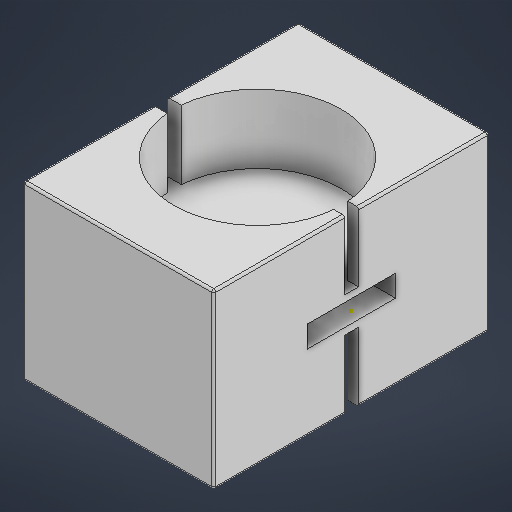
# Autodesk Inventor part: Base_Casing_A0645_v2
Saved by Autodesk Inventor 2026.1 (Build 301233020, 233B)
## iProperties
Created: 2025-09-05
Part Number: Base_Casing_A0645_v2
Material: Generic
Document SubType Name: Modeling
Designer: usman
Density: 1 g/cm^3
Appearance: Default
Author: usman
Autodesk Inventor part; units mm, degrees
ref_plane "YZ Plane" through (0, 0, 0) normal (1, 0, 0) x (0, 1, 0)
ref_plane "XZ Plane" through (0, 0, 0) normal (0, 1, 0) x (-1, 0, 0)
ref_plane "XY Plane" through (0, 0, 0) normal (0, 0, 1) x (1, 0, 0)
sketch "Sketch1" plane through (0, 0, 0) normal (1, 0, 0) x (0, 1, 0)
  line L0 (-39.75, 63.5) -> (39.75, 63.5)
  line L1 (39.75, 63.5) -> (39.75, -63.5)
  line L2 (39.75, -63.5) -> (-39.75, -63.5)
  line L3 (-39.75, -63.5) -> (-39.75, 63.5)
  line L4 (-39.75, 63.5) -> (39.75, -63.5) construction
  line L5 (39.75, 63.5) -> (-39.75, -63.5) construction
  point P0 (0, 0)
  dimension "d0" = 79.5
  constraints: 12 end point, 2 midpoint, 2 parallel, 1 horizontal, 1 perpendicular
  measures "d0" distance of L1.end L2.end
extrude "Extrusion1" add sketch "Sketch1" along normal blind 88
sketch "Sketch2" plane through (88, 0, 0) normal (1, 0, 0) x (0, 0, -1)
  line L0 (-20.32, -5) -> (20.32, -5)
  line L1 (20.32, -5) -> (20.32, 5)
  line L2 (20.32, 5) -> (-20.32, 5)
  line L3 (-20.32, 5) -> (-20.32, -5)
  line L4 (-20.32, -5) -> (20.32, 5) construction
  line L5 (20.32, -5) -> (-20.32, 5) construction
  point P0 (0, 0)
  dimension "d4" = 10
  dimension "d5" = 40.64
  constraints: 12 end point, 2 midpoint, 2 parallel, 1 horizontal, 1 perpendicular
  measures "d4" distance of L0.end L1.end
  measures "d5" distance of L1.end L2.end
extrude "Extrusion2" cut sketch "Sketch2" against normal through all
sketch "Sketch3" plane through (88, 0, 0) normal (1, 0, 0) x (0, 0, -1)
  point P0 (0, 0)
sketch "Sketch4" plane through (0, 39.75, 63.5) normal (0, 1, 0) x (1, 0, 0)
  line L0 (82.3836, 27.6051) -> (7, 99.3949) construction
  line L1 (7, 27.6051) -> (82.3836, 99.3949) construction
  line L2 (0, 127) -> (0, 0) projected
  line L3 (0, 127) -> (88, 127) projected
  circle A0 centre (44.6918, 63.5) radius 38.5
  point P0 (0, 63.5)
  dimension "d23" = 77
  dimension "d24" = 127
  dimension "d25" = 63.5
  constraints: 4 end point, 2 midpoint, 1 centre point, 1 coincident
  measures "d23" diameter of A0
  measures "d24" distance of L2.start L2.end
  measures "d25" vertical distance of point (44.692, 63.5) L2.end
extrude "Extrusion3" cut sketch "Sketch4" against normal blind 31.7
mirror "Mirror1" about plane through (0, 0, 0) normal (0, 1, 0) of "Extrusion3"
sketch "Sketch5" plane through (0, 0, 0) normal (-1, 0, 0) x (0, 0, 1)
  line L0 (-63.5, 39.75) -> (63.5, 39.75) projected
  line L1 (-3.25, 8.05) -> (3.25, 8.05)
  line L2 (3.25, 8.05) -> (3.25, 39.75)
  line L3 (3.25, 39.75) -> (-3.25, 39.75)
  line L4 (-3.25, 39.75) -> (-3.25, 8.05)
  line L5 (-3.25, 8.05) -> (3.25, 39.75) construction
  line L6 (3.25, 8.05) -> (-3.25, 39.75) construction
  point P0 (0, 0)
  point P1 (0, 23.9)
  point P2 (-3.25, 39.75)
  dimension "d12" = 3.25
  dimension "d13" = 31.7
  constraints: 12 end point, 2 midpoint, 2 parallel, 1 horizontal, 1 perpendicular, 1 point on line
  measures "d12" distance from line of point (0, 23.9) L2
  measures "d13" distance of L1.end L2.end
extrude "Extrusion4" cut sketch "Sketch5" against normal through all
mirror "Mirror2" about plane through (0, 0, 0) normal (0, 1, 0) of "Extrusion4"
sketch "Sketch6" plane through (0, 0, 0) normal (-1, 0, 0) x (0, 0, 1)
  line L0 (-53.1221, 38.1768) -> (-13.6279, 38.1768) construction
  line L1 (-13.6279, 38.1768) -> (-13.6279, 7.4202) construction
  line L2 (-13.6279, 7.4202) -> (-53.1221, 7.4202) construction
  line L3 (-53.1221, 7.4202) -> (-53.1221, 38.1768) construction
  line L4 (-63.5, 39.75) -> (-3.25, 39.75) projected
  line L5 (-42.524, 25.8134) -> (-42.524, 31.9094)
  line L6 (-42.524, 31.9094) -> (-41.5692, 31.9094)
  spline S0 degree 2 poles (-41.5692, 31.9094) (-40.7349, 31.9094) (-40.348, 31.8039) knots 0 0 0 1 1 1
  spline S1 degree 2 poles (-40.348, 31.8039) (-39.8052, 31.6581) (-39.1569, 30.8691) (-39.1569, 30.3364) knots 0 0 0 1 2 2 2
  spline S2 degree 2 poles (-39.1569, 30.3364) (-39.1569, 29.9846) (-39.4484, 29.4167) (-39.7801, 29.1705) knots 0 0 0 1 2 2 2
  spline S3 degree 2 poles (-39.7801, 29.1705) (-39.2222, 28.9091) (-38.7096, 28.1252) (-38.7096, 27.5924) knots 0 0 0 1 2 2 2
  spline S4 degree 2 poles (-38.7096, 27.5924) (-38.7096, 27.0748) (-39.2423, 26.2305) (-40.0766, 25.8134) (-40.8153, 25.8134) knots 0 0 0 1 2 3 3 3
  line L7 (-40.8153, 25.8134) -> (-42.524, 25.8134)
  line L8 (-41.3631, 28.482) -> (-41.3631, 26.919)
  line L9 (-41.3631, 26.919) -> (-41.0716, 26.919)
  spline S5 degree 2 poles (-41.0716, 26.919) (-40.353, 26.919) (-39.8504, 27.2859) (-39.8504, 27.6327) knots 0 0 0 1 2 2 2
  spline S6 degree 2 poles (-39.8504, 27.6327) (-39.8504, 28.0246) (-40.4384, 28.482) (-41.1219, 28.482) knots 0 0 0 1 2 2 2
  line L10 (-41.1219, 28.482) -> (-41.3631, 28.482)
  line L11 (-41.3631, 30.8038) -> (-41.3631, 29.5172)
  line L12 (-41.3631, 29.5172) -> (-41.1118, 29.5172)
  spline S7 degree 2 poles (-41.1118, 29.5172) (-40.6897, 29.5172) (-40.2776, 29.8741) (-40.2776, 30.1806) knots 0 0 0 1 2 2 2
  spline S8 degree 2 poles (-40.2776, 30.1806) (-40.2776, 30.4671) (-40.6646, 30.8038) (-41.0666, 30.8038) knots 0 0 0 1 2 2 2
  line L13 (-41.0666, 30.8038) -> (-41.3631, 30.8038)
  line L14 (-34.3977, 30.3213) -> (-33.267, 30.3213)
  line L15 (-33.267, 30.3213) -> (-33.267, 25.8134)
  line L16 (-33.267, 25.8134) -> (-34.3977, 25.8134)
  line L17 (-34.3977, 25.8134) -> (-34.3977, 26.2908)
  spline S9 degree 2 poles (-34.3977, 26.2908) (-34.7294, 25.9742) (-35.3928, 25.6978) (-35.7848, 25.6978) knots 0 0 0 1 2 2 2
  spline S10 degree 2 poles (-35.7848, 25.6978) (-36.6542, 25.6978) (-37.9307, 27.0547) (-37.9307, 28.0598) knots 0 0 0 1 2 2 2
  spline S11 degree 2 poles (-37.9307, 28.0598) (-37.9307, 29.1051) (-36.6994, 30.4369) (-35.8149, 30.4369) knots 0 0 0 1 2 2 2
  spline S12 degree 2 poles (-35.8149, 30.4369) (-35.4129, 30.4369) (-34.6992, 30.1304) (-34.3977, 29.8238) knots 0 0 0 1 2 2 2
  line L18 (-34.3977, 29.8238) -> (-34.3977, 30.3213)
  spline S13 degree 2 poles (-35.5888, 29.3916) (-36.1114, 29.3916) (-36.8049, 28.6528) (-36.8049, 28.0699) knots 0 0 0 1 2 2 2
  spline S14 degree 2 poles (-36.8049, 28.0699) (-36.8049, 27.4869) (-36.0963, 26.7331) (-35.5837, 26.7331) knots 0 0 0 1 2 2 2
  spline S15 degree 2 poles (-35.5837, 26.7331) (-35.051, 26.7331) (-34.3474, 27.4769) (-34.3474, 28.0749) knots 0 0 0 1 2 2 2
  spline S16 degree 2 poles (-34.3474, 28.0749) (-34.3474, 28.6629) (-35.051, 29.3916) (-35.5888, 29.3916) knots 0 0 0 1 2 2 2
  line L19 (-29.3671, 29.6881) -> (-30.0657, 28.9896)
  spline S17 degree 2 poles (-30.0657, 28.9896) (-30.4878, 29.4117) (-30.8346, 29.4117) knots 0 0 0 1 1 1
  spline S18 degree 2 poles (-30.8346, 29.4117) (-31.0256, 29.4117) (-31.2417, 29.2509) (-31.2417, 29.1303) knots 0 0 0 1 2 2 2
  spline S19 degree 2 poles (-31.2417, 29.1303) (-31.2417, 29.0398) (-31.106, 28.884) (-30.8346, 28.7534) knots 0 0 0 1 2 2 2
  line L20 (-30.8346, 28.7534) -> (-30.4225, 28.5473)
  spline S20 degree 2 poles (-30.4225, 28.5473) (-29.7692, 28.2257) (-29.2817, 27.5522) (-29.2817, 27.0999) knots 0 0 0 1 2 2 2
  spline S21 degree 2 poles (-29.2817, 27.0999) (-29.2817, 26.5019) (-30.1612, 25.6978) (-30.9049, 25.6978) knots 0 0 0 1 2 2 2
  spline S22 degree 2 poles (-30.9049, 25.6978) (-31.8899, 25.6978) (-32.4779, 26.4667) knots 0 0 0 1 1 1
  line L21 (-32.4779, 26.4667) -> (-31.7844, 27.2256)
  spline S23 degree 2 poles (-31.7844, 27.2256) (-31.5834, 26.9944) (-31.0507, 26.708) (-30.8446, 26.708) knots 0 0 0 1 2 2 2
  spline S24 degree 2 poles (-30.8446, 26.708) (-30.6185, 26.708) (-30.3471, 26.924) (-30.3471, 27.0648) knots 0 0 0 1 2 2 2
  spline S25 degree 2 poles (-30.3471, 27.0648) (-30.3471, 27.3261) (-30.8396, 27.5723) knots 0 0 0 1 1 1
  line L22 (-30.8396, 27.5723) -> (-31.2215, 27.7633)
  spline S26 degree 2 poles (-31.2215, 27.7633) (-32.3121, 28.3161) (-32.3121, 29.1453) knots 0 0 0 1 1 1
  spline S27 degree 2 poles (-32.3121, 29.1453) (-32.3121, 29.6781) (-31.4879, 30.4369) (-30.8497, 30.4369) knots 0 0 0 1 2 2 2
  spline S28 degree 2 poles (-30.8497, 30.4369) (-30.4074, 30.4369) (-29.6335, 30.0499) (-29.3671, 29.6881) knots 0 0 0 1 2 2 2
  line L23 (-23.8742, 27.7432) -> (-27.5026, 27.7432)
  spline S29 degree 2 poles (-27.5026, 27.7432) (-27.4222, 27.2608) (-26.7388, 26.6929) (-26.2111, 26.6929) knots 0 0 0 1 2 2 2
  spline S30 degree 2 poles (-26.2111, 26.6929) (-25.5778, 26.6929) (-25.1205, 27.1351) knots 0 0 0 1 1 1
  line L24 (-25.1205, 27.1351) -> (-24.1707, 26.6878)
  spline S31 degree 2 poles (-24.1707, 26.6878) (-24.5275, 26.1853) (-25.5226, 25.6978) (-26.206, 25.6978) knots 0 0 0 1 2 2 2
  spline S32 degree 2 poles (-26.206, 25.6978) (-27.2664, 25.6978) (-28.5982, 27.0346) (-28.5982, 28.0447) knots 0 0 0 1 2 2 2
  spline S33 degree 2 poles (-28.5982, 28.0447) (-28.5982, 29.075) (-27.2664, 30.4369) (-26.2664, 30.4369) knots 0 0 0 1 2 2 2
  spline S34 degree 2 poles (-26.2664, 30.4369) (-25.2009, 30.4369) (-23.8692, 29.075) (-23.8692, 27.9593) knots 0 0 0 1 2 2 2
  line L25 (-23.8692, 27.9593) -> (-23.8742, 27.7432)
  spline S35 degree 2 poles (-25.0049, 28.6327) (-25.1155, 29.0097) (-25.7738, 29.477) (-26.2111, 29.477) knots 0 0 0 1 2 2 2
  spline S36 degree 2 poles (-26.2111, 29.477) (-26.6835, 29.477) (-27.0403, 29.2157) knots 0 0 0 1 1 1
  spline S37 degree 2 poles (-27.0403, 29.2157) (-27.2614, 29.0499) (-27.4524, 28.6327) knots 0 0 0 1 1 1
  line L26 (-27.4524, 28.6327) -> (-25.0049, 28.6327)
  line L27 (-48.0471, 21.5476) -> (-46.9214, 21.5476)
  line L28 (-46.9214, 21.5476) -> (-45.5042, 17.296)
  line L29 (-45.5042, 17.296) -> (-44.0769, 21.5476)
  line L30 (-44.0769, 21.5476) -> (-42.9512, 21.5476)
  line L31 (-42.9512, 21.5476) -> (-41.931, 15.4516)
  line L32 (-41.931, 15.4516) -> (-43.0517, 15.4516)
  line L33 (-43.0517, 15.4516) -> (-43.7, 19.3012)
  line L34 (-43.7, 19.3012) -> (-44.9966, 15.4516)
  line L35 (-44.9966, 15.4516) -> (-46.0218, 15.4516)
  line L36 (-46.0218, 15.4516) -> (-47.3033, 19.3012)
  line L37 (-47.3033, 19.3012) -> (-47.9717, 15.4516)
  line L38 (-47.9717, 15.4516) -> (-49.1025, 15.4516)
  line L39 (-49.1025, 15.4516) -> (-48.0471, 21.5476)
  line L40 (-37.795, 19.9595) -> (-36.6642, 19.9595)
  line L41 (-36.6642, 19.9595) -> (-36.6642, 15.4516)
  line L42 (-36.6642, 15.4516) -> (-37.795, 15.4516)
  line L43 (-37.795, 15.4516) -> (-37.795, 15.929)
  spline S38 degree 2 poles (-37.795, 15.929) (-38.1267, 15.6124) (-38.79, 15.336) (-39.182, 15.336) knots 0 0 0 1 2 2 2
  spline S39 degree 2 poles (-39.182, 15.336) (-40.0515, 15.336) (-41.3279, 16.6929) (-41.3279, 17.698) knots 0 0 0 1 2 2 2
  spline S40 degree 2 poles (-41.3279, 17.698) (-41.3279, 18.7433) (-40.0967, 20.0751) (-39.2122, 20.0751) knots 0 0 0 1 2 2 2
  spline S41 degree 2 poles (-39.2122, 20.0751) (-38.8101, 20.0751) (-38.0965, 19.7685) (-37.795, 19.462) knots 0 0 0 1 2 2 2
  line L44 (-37.795, 19.462) -> (-37.795, 19.9595)
  spline S42 degree 2 poles (-38.986, 19.0298) (-39.5087, 19.0298) (-40.2022, 18.291) (-40.2022, 17.7081) knots 0 0 0 1 2 2 2
  spline S43 degree 2 poles (-40.2022, 17.7081) (-40.2022, 17.1251) (-39.4936, 16.3713) (-38.981, 16.3713) knots 0 0 0 1 2 2 2
  spline S44 degree 2 poles (-38.981, 16.3713) (-38.4483, 16.3713) (-37.7447, 17.115) (-37.7447, 17.7131) knots 0 0 0 1 2 2 2
  spline S45 degree 2 poles (-37.7447, 17.7131) (-37.7447, 18.3011) (-38.4483, 19.0298) (-38.986, 19.0298) knots 0 0 0 1 2 2 2
  line L45 (-32.1915, 19.9595) -> (-31.0607, 19.9595)
  line L46 (-31.0607, 19.9595) -> (-31.0607, 16.0999)
  spline S46 degree 2 poles (-31.0607, 16.0999) (-31.0607, 14.9541) (-31.5231, 14.4163) knots 0 0 0 1 1 1
  spline S47 degree 2 poles (-31.5231, 14.4163) (-32.1362, 13.6876) (-33.3825, 13.6876) knots 0 0 0 1 1 1
  spline S48 degree 2 poles (-33.3825, 13.6876) (-34.0459, 13.6876) (-34.9455, 14.0193) (-35.5687, 14.6626) (-35.7194, 15.1199) knots 0 0 0 1 2 3 3 3
  line L47 (-35.7194, 15.1199) -> (-34.4731, 15.1199)
  spline S49 degree 2 poles (-34.4731, 15.1199) (-34.3072, 14.9289) (-33.7846, 14.738) (-33.4278, 14.738) knots 0 0 0 1 2 2 2
  spline S50 degree 2 poles (-33.4278, 14.738) (-32.9755, 14.738) (-32.4176, 15.0194) (-32.1915, 15.4667) (-32.1915, 16.0145) knots 0 0 0 1 2 3 3 3
  spline S51 degree 2 poles (-32.1915, 16.0145) (-32.488, 15.7129) (-33.1413, 15.4516) (-33.5584, 15.4516) knots 0 0 0 1 2 2 2
  spline S52 degree 2 poles (-33.5584, 15.4516) (-34.463, 15.4516) (-35.7144, 16.7633) (-35.7144, 17.7633) knots 0 0 0 1 2 2 2
  spline S53 degree 2 poles (-35.7144, 17.7633) (-35.7144, 18.8388) (-35.051, 19.4871) knots 0 0 0 1 1 1
  spline S54 degree 2 poles (-35.051, 19.4871) (-34.453, 20.0751) (-33.6187, 20.0751) knots 0 0 0 1 1 1
  spline S55 degree 2 poles (-33.6187, 20.0751) (-33.2318, 20.0751) (-32.5382, 19.7886) (-32.1915, 19.462) knots 0 0 0 1 2 2 2
  line L48 (-32.1915, 19.462) -> (-32.1915, 19.9595)
  spline S56 degree 2 poles (-33.3574, 19.0197) (-33.8951, 19.0197) (-34.5887, 18.3011) (-34.5887, 17.7583) knots 0 0 0 1 2 2 2
  spline S57 degree 2 poles (-34.5887, 17.7583) (-34.5887, 17.1955) (-33.875, 16.4768) (-33.3373, 16.4768) knots 0 0 0 1 2 2 2
  spline S58 degree 2 poles (-33.3373, 16.4768) (-32.8146, 16.4768) (-32.1312, 17.1804) (-32.1312, 17.7533) knots 0 0 0 1 2 2 2
  spline S59 degree 2 poles (-32.1312, 17.7533) (-32.1312, 18.3162) (-32.8197, 19.0197) (-33.3574, 19.0197) knots 0 0 0 1 2 2 2
  line L49 (-29.9149, 19.9595) -> (-28.7842, 19.9595)
  line L50 (-28.7842, 19.9595) -> (-28.7842, 19.4972)
  spline S60 degree 2 poles (-28.7842, 19.4972) (-28.3972, 19.8238) (-27.774, 20.0751) (-27.4474, 20.0751) knots 0 0 0 1 2 2 2
  spline S61 degree 2 poles (-27.4474, 20.0751) (-26.7739, 20.0751) (-26.3066, 19.6077) knots 0 0 0 1 1 1
  spline S62 degree 2 poles (-26.3066, 19.6077) (-25.9146, 19.2107) (-25.9146, 18.4317) knots 0 0 0 1 1 1
  line L51 (-25.9146, 18.4317) -> (-25.9146, 15.4516)
  line L52 (-25.9146, 15.4516) -> (-27.0353, 15.4516)
  line L53 (-27.0353, 15.4516) -> (-27.0353, 17.4266)
  spline S63 degree 2 poles (-27.0353, 17.4266) (-27.0353, 18.2307) (-27.181, 18.7634) (-27.5378, 19.0398) (-27.8042, 19.0398) knots 0 0 0 1 2 3 3 3
  spline S64 degree 2 poles (-27.8042, 19.0398) (-28.1459, 19.0398) (-28.6384, 18.5825) (-28.7339, 18.1754) knots 0 0 0 1 2 2 2
  spline S65 degree 2 poles (-28.7339, 18.1754) (-28.7842, 17.9644) (-28.7842, 17.2608) knots 0 0 0 1 1 1
  line L54 (-28.7842, 17.2608) -> (-28.7842, 15.4516)
  line L55 (-28.7842, 15.4516) -> (-29.9149, 15.4516)
  line L56 (-29.9149, 15.4516) -> (-29.9149, 19.9595)
  line L57 (-20.306, 17.3814) -> (-23.9345, 17.3814)
  spline S66 degree 2 poles (-23.9345, 17.3814) (-23.8541, 16.8989) (-23.1706, 16.3311) (-22.6429, 16.3311) knots 0 0 0 1 2 2 2
  spline S67 degree 2 poles (-22.6429, 16.3311) (-22.0097, 16.3311) (-21.5524, 16.7733) knots 0 0 0 1 1 1
  line L58 (-21.5524, 16.7733) -> (-20.6025, 16.326)
  spline S68 degree 2 poles (-20.6025, 16.326) (-20.9594, 15.8235) (-21.9544, 15.336) (-22.6379, 15.336) knots 0 0 0 1 2 2 2
  spline S69 degree 2 poles (-22.6379, 15.336) (-23.6983, 15.336) (-25.0301, 16.6728) (-25.0301, 17.6829) knots 0 0 0 1 2 2 2
  spline S70 degree 2 poles (-25.0301, 17.6829) (-25.0301, 18.7132) (-23.6983, 20.0751) (-22.6982, 20.0751) knots 0 0 0 1 2 2 2
  spline S71 degree 2 poles (-22.6982, 20.0751) (-21.6328, 20.0751) (-20.301, 18.7132) (-20.301, 17.5975) knots 0 0 0 1 2 2 2
  line L59 (-20.301, 17.5975) -> (-20.306, 17.3814)
  spline S72 degree 2 poles (-21.4368, 18.2709) (-21.5474, 18.6478) (-22.2057, 19.1152) (-22.6429, 19.1152) knots 0 0 0 1 2 2 2
  spline S73 degree 2 poles (-22.6429, 19.1152) (-23.1153, 19.1152) (-23.4721, 18.8539) knots 0 0 0 1 1 1
  spline S74 degree 2 poles (-23.4721, 18.8539) (-23.6933, 18.688) (-23.8842, 18.2709) knots 0 0 0 1 1 1
  line L60 (-23.8842, 18.2709) -> (-21.4368, 18.2709)
  line L61 (-19.2507, 21.623) -> (-18.1199, 21.623)
  line L62 (-18.1199, 21.623) -> (-18.1199, 19.9595)
  line L63 (-18.1199, 19.9595) -> (-17.4465, 19.9595)
  line L64 (-17.4465, 19.9595) -> (-17.4465, 18.9846)
  line L65 (-17.4465, 18.9846) -> (-18.1199, 18.9846)
  line L66 (-18.1199, 18.9846) -> (-18.1199, 15.4516)
  line L67 (-18.1199, 15.4516) -> (-19.2507, 15.4516)
  line L68 (-19.2507, 15.4516) -> (-19.2507, 18.9846)
  line L69 (-19.2507, 18.9846) -> (-19.8286, 18.9846)
  line L70 (-19.8286, 18.9846) -> (-19.8286, 19.9595)
  line L71 (-19.8286, 19.9595) -> (-19.2507, 19.9595)
  line L72 (-19.2507, 19.9595) -> (-19.2507, 21.623)
  point P0 (0, 0)
  point P1 (-33.375, 39.75)
  point P2 (-33.375, 38.1768)
  dimension "d0" = 79.5
  dimension "d26" = 0
  constraints: 2 midpoint, 2 other
  measures "d26" horizontal distance of point (-33.375, 39.75) point (-33.375, 38.177)
sketch "Sketch7" plane through (0, 0, 0) normal (-1, 0, 0) x (0, 0, 1)
  line L0 (14.6764, 37.9215) -> (52.0736, 37.9215) construction
  line L1 (52.0736, 37.9215) -> (52.0736, 6.8154) construction
  line L2 (52.0736, 6.8154) -> (14.6764, 6.8154) construction
  line L3 (14.6764, 6.8154) -> (14.6764, 37.9215) construction
  line L4 (-51.8647, -8.5629) -> (-14.8853, -8.5629) construction
  line L5 (-14.8853, -8.5629) -> (-14.8853, -37.9215) construction
  line L6 (-14.8853, -37.9215) -> (-51.8647, -37.9215) construction
  line L7 (-51.8647, -37.9215) -> (-51.8647, -8.5629) construction
  line L8 (3.25, 39.75) -> (63.5, 39.75) projected
  line L9 (-3.25, -39.75) -> (-63.5, -39.75) projected
  line L10 (25.3266, 25.0873) -> (24.5175, 24.3133)
  spline S0 degree 2 poles (24.5175, 24.3133) (23.6882, 25.1878) (22.653, 25.1878) knots 0 0 0 1 1 1
  spline S1 degree 2 poles (22.653, 25.1878) (21.7785, 25.1878) (20.5824, 23.9967) (20.5824, 23.1223) knots 0 0 0 1 2 2 2
  spline S2 degree 2 poles (20.5824, 23.1223) (20.5824, 22.5142) (21.1101, 21.5694) (22.0801, 21.0316) (22.6731, 21.0316) knots 0 0 0 1 2 3 3 3
  spline S3 degree 2 poles (22.6731, 21.0316) (23.1756, 21.0316) (24.0149, 21.4085) (24.5175, 21.9061) knots 0 0 0 1 2 2 2
  line L11 (24.5175, 21.9061) -> (25.3014, 21.0869)
  spline S4 degree 2 poles (25.3014, 21.0869) (24.628, 20.4235) (23.4269, 19.916) (22.653, 19.916) knots 0 0 0 1 2 2 2
  spline S5 degree 2 poles (22.653, 19.916) (21.2307, 19.916) (19.4215, 21.7151) (19.4215, 23.1273) knots 0 0 0 1 2 2 2
  spline S6 degree 2 poles (19.4215, 23.1273) (19.4215, 24.0369) (20.2457, 25.4541) (21.7836, 26.3135) (22.6681, 26.3135) knots 0 0 0 1 2 3 3 3
  spline S7 degree 2 poles (22.6681, 26.3135) (23.4269, 26.3135) (24.819, 25.6752) (25.3266, 25.0873) knots 0 0 0 1 2 2 2
  line L12 (29.548, 24.5746) -> (30.6788, 24.5746)
  line L13 (30.6788, 24.5746) -> (30.6788, 20.0667)
  line L14 (30.6788, 20.0667) -> (29.548, 20.0667)
  line L15 (29.548, 20.0667) -> (29.548, 20.5442)
  spline S8 degree 2 poles (29.548, 20.5442) (29.2164, 20.2275) (28.553, 19.9511) (28.161, 19.9511) knots 0 0 0 1 2 2 2
  spline S9 degree 2 poles (28.161, 19.9511) (27.2916, 19.9511) (26.0151, 21.308) (26.0151, 22.3131) knots 0 0 0 1 2 2 2
  spline S10 degree 2 poles (26.0151, 22.3131) (26.0151, 23.3585) (27.2463, 24.6902) (28.1308, 24.6902) knots 0 0 0 1 2 2 2
  spline S11 degree 2 poles (28.1308, 24.6902) (28.5329, 24.6902) (29.2465, 24.3837) (29.548, 24.0771) knots 0 0 0 1 2 2 2
  line L16 (29.548, 24.0771) -> (29.548, 24.5746)
  spline S12 degree 2 poles (28.357, 23.6449) (27.8343, 23.6449) (27.1408, 22.9062) (27.1408, 22.3232) knots 0 0 0 1 2 2 2
  spline S13 degree 2 poles (27.1408, 22.3232) (27.1408, 21.7402) (27.8494, 20.9864) (28.362, 20.9864) knots 0 0 0 1 2 2 2
  spline S14 degree 2 poles (28.362, 20.9864) (28.8947, 20.9864) (29.5983, 21.7302) (29.5983, 22.3282) knots 0 0 0 1 2 2 2
  spline S15 degree 2 poles (29.5983, 22.3282) (29.5983, 22.9162) (28.8947, 23.6449) (28.357, 23.6449) knots 0 0 0 1 2 2 2
  line L17 (34.5786, 23.9414) -> (33.8801, 23.2429)
  spline S16 degree 2 poles (33.8801, 23.2429) (33.4579, 23.665) (33.1112, 23.665) knots 0 0 0 1 1 1
  spline S17 degree 2 poles (33.1112, 23.665) (32.9202, 23.665) (32.7041, 23.5042) (32.7041, 23.3836) knots 0 0 0 1 2 2 2
  spline S18 degree 2 poles (32.7041, 23.3836) (32.7041, 23.2931) (32.8398, 23.1373) (33.1112, 23.0067) knots 0 0 0 1 2 2 2
  line L18 (33.1112, 23.0067) -> (33.5233, 22.8006)
  spline S19 degree 2 poles (33.5233, 22.8006) (34.1766, 22.479) (34.6641, 21.8056) (34.6641, 21.3533) knots 0 0 0 1 2 2 2
  spline S20 degree 2 poles (34.6641, 21.3533) (34.6641, 20.7552) (33.7846, 19.9511) (33.0408, 19.9511) knots 0 0 0 1 2 2 2
  spline S21 degree 2 poles (33.0408, 19.9511) (32.0558, 19.9511) (31.4678, 20.72) knots 0 0 0 1 1 1
  line L19 (31.4678, 20.72) -> (32.1613, 21.4789)
  spline S22 degree 2 poles (32.1613, 21.4789) (32.3624, 21.2477) (32.8951, 20.9613) (33.1011, 20.9613) knots 0 0 0 1 2 2 2
  spline S23 degree 2 poles (33.1011, 20.9613) (33.3273, 20.9613) (33.5986, 21.1774) (33.5986, 21.3181) knots 0 0 0 1 2 2 2
  spline S24 degree 2 poles (33.5986, 21.3181) (33.5986, 21.5794) (33.1061, 21.8257) knots 0 0 0 1 1 1
  line L20 (33.1061, 21.8257) -> (32.7242, 22.0166)
  spline S25 degree 2 poles (32.7242, 22.0166) (31.6336, 22.5695) (31.6336, 23.3987) knots 0 0 0 1 1 1
  spline S26 degree 2 poles (31.6336, 23.3987) (31.6336, 23.9314) (32.4578, 24.6902) (33.0961, 24.6902) knots 0 0 0 1 2 2 2
  spline S27 degree 2 poles (33.0961, 24.6902) (33.5383, 24.6902) (34.3123, 24.3033) (34.5786, 23.9414) knots 0 0 0 1 2 2 2
  line L21 (35.433, 24.5746) -> (36.5637, 24.5746)
  line L22 (36.5637, 24.5746) -> (36.5637, 20.0667)
  line L23 (36.5637, 20.0667) -> (35.433, 20.0667)
  line L24 (35.433, 20.0667) -> (35.433, 24.5746)
  spline S28 degree 2 poles (35.9958, 26.4341) (36.2923, 26.4341) (36.7195, 26.0019) (36.7195, 25.6953) knots 0 0 0 1 2 2 2
  spline S29 degree 2 poles (36.7195, 25.6953) (36.7195, 25.3938) (36.2974, 24.9666) (36.0059, 24.9666) knots 0 0 0 1 2 2 2
  spline S30 degree 2 poles (36.0059, 24.9666) (35.7043, 24.9666) (35.2772, 25.4039) (35.2772, 25.7104) knots 0 0 0 1 2 2 2
  spline S31 degree 2 poles (35.2772, 25.7104) (35.2772, 26.012) (35.6993, 26.4341) (35.9958, 26.4341) knots 0 0 0 1 2 2 2
  line L25 (37.594, 24.5746) -> (38.7247, 24.5746)
  line L26 (38.7247, 24.5746) -> (38.7247, 24.1123)
  spline S32 degree 2 poles (38.7247, 24.1123) (39.1117, 24.439) (39.7348, 24.6902) (40.0615, 24.6902) knots 0 0 0 1 2 2 2
  spline S33 degree 2 poles (40.0615, 24.6902) (40.7349, 24.6902) (41.2023, 24.2229) knots 0 0 0 1 1 1
  spline S34 degree 2 poles (41.2023, 24.2229) (41.5943, 23.8258) (41.5943, 23.0469) knots 0 0 0 1 1 1
  line L27 (41.5943, 23.0469) -> (41.5943, 20.0667)
  line L28 (41.5943, 20.0667) -> (40.4736, 20.0667)
  line L29 (40.4736, 20.0667) -> (40.4736, 22.0418)
  spline S35 degree 2 poles (40.4736, 22.0418) (40.4736, 22.8459) (40.3279, 23.3786) (39.971, 23.655) (39.7047, 23.655) knots 0 0 0 1 2 3 3 3
  spline S36 degree 2 poles (39.7047, 23.655) (39.363, 23.655) (38.8704, 23.1976) (38.775, 22.7906) knots 0 0 0 1 2 2 2
  spline S37 degree 2 poles (38.775, 22.7906) (38.7247, 22.5795) (38.7247, 21.8759) knots 0 0 0 1 1 1
  line L30 (38.7247, 21.8759) -> (38.7247, 20.0667)
  line L31 (38.7247, 20.0667) -> (37.594, 20.0667)
  line L32 (37.594, 20.0667) -> (37.594, 24.5746)
  line L33 (46.0168, 24.5746) -> (47.1475, 24.5746)
  line L34 (47.1475, 24.5746) -> (47.1475, 20.715)
  spline S38 degree 2 poles (47.1475, 20.715) (47.1475, 19.5692) (46.6852, 19.0315) knots 0 0 0 1 1 1
  spline S39 degree 2 poles (46.6852, 19.0315) (46.0721, 18.3028) (44.8257, 18.3028) knots 0 0 0 1 1 1
  spline S40 degree 2 poles (44.8257, 18.3028) (44.1624, 18.3028) (43.2628, 18.6344) (42.6396, 19.2777) (42.4888, 19.735) knots 0 0 0 1 2 3 3 3
  line L35 (42.4888, 19.735) -> (43.7352, 19.735)
  spline S41 degree 2 poles (43.7352, 19.735) (43.901, 19.5441) (44.4237, 19.3531) (44.7805, 19.3531) knots 0 0 0 1 2 2 2
  spline S42 degree 2 poles (44.7805, 19.3531) (45.2328, 19.3531) (45.7906, 19.6345) (46.0168, 20.0818) (46.0168, 20.6296) knots 0 0 0 1 2 3 3 3
  spline S43 degree 2 poles (46.0168, 20.6296) (45.7203, 20.3281) (45.067, 20.0667) (44.6498, 20.0667) knots 0 0 0 1 2 2 2
  spline S44 degree 2 poles (44.6498, 20.0667) (43.7452, 20.0667) (42.4939, 21.3784) (42.4939, 22.3785) knots 0 0 0 1 2 2 2
  spline S45 degree 2 poles (42.4939, 22.3785) (42.4939, 23.4539) (43.1572, 24.1022) knots 0 0 0 1 1 1
  spline S46 degree 2 poles (43.1572, 24.1022) (43.7553, 24.6902) (44.5895, 24.6902) knots 0 0 0 1 1 1
  spline S47 degree 2 poles (44.5895, 24.6902) (44.9765, 24.6902) (45.67, 24.4038) (46.0168, 24.0771) knots 0 0 0 1 2 2 2
  line L36 (46.0168, 24.0771) -> (46.0168, 24.5746)
  spline S48 degree 2 poles (44.8509, 23.6349) (44.3131, 23.6349) (43.6196, 22.9162) (43.6196, 22.3735) knots 0 0 0 1 2 2 2
  spline S49 degree 2 poles (43.6196, 22.3735) (43.6196, 21.8106) (44.3332, 21.0919) (44.871, 21.0919) knots 0 0 0 1 2 2 2
  spline S50 degree 2 poles (44.871, 21.0919) (45.3936, 21.0919) (46.0771, 21.7955) (46.0771, 22.3684) knots 0 0 0 1 2 2 2
  spline S51 degree 2 poles (46.0771, 22.3684) (46.0771, 22.9313) (45.3886, 23.6349) (44.8509, 23.6349) knots 0 0 0 1 2 2 2
  line L37 (-50.6001, -20.1942) -> (-49.4191, -20.1942)
  line L38 (-49.4191, -20.1942) -> (-47.0772, -26.2902)
  line L39 (-47.0772, -26.2902) -> (-48.2833, -26.2902)
  line L40 (-48.2833, -26.2902) -> (-48.7607, -25.0338)
  line L41 (-48.7607, -25.0338) -> (-51.2484, -25.0338)
  line L42 (-51.2484, -25.0338) -> (-51.7409, -26.2902)
  line L43 (-51.7409, -26.2902) -> (-52.947, -26.2902)
  line L44 (-52.947, -26.2902) -> (-50.6001, -20.1942)
  line L45 (-50.0021, -21.8124) -> (-50.8212, -23.9031)
  line L46 (-50.8212, -23.9031) -> (-49.1929, -23.9031)
  line L47 (-49.1929, -23.9031) -> (-50.0021, -21.8124)
  spline S52 degree 2 poles (-44.5192, -20.0434) (-43.8508, -20.0434) (-42.8859, -20.6968) (-42.3582, -22.0436) (-42.3582, -23.2447) knots 0 0 0 1 2 3 3 3
  spline S53 degree 2 poles (-42.3582, -23.2447) (-42.3582, -24.4559) (-42.8909, -25.8077) (-43.7955, -26.441) (-44.484, -26.441) knots 0 0 0 1 2 3 3 3
  spline S54 degree 2 poles (-44.484, -26.441) (-45.1725, -26.441) (-46.1072, -25.8027) (-46.64, -24.5011) (-46.64, -23.3) knots 0 0 0 1 2 3 3 3
  spline S55 degree 2 poles (-46.64, -23.3) (-46.64, -21.6265) (-46.1223, -20.8726) knots 0 0 0 1 1 1
  spline S56 degree 2 poles (-46.1223, -20.8726) (-45.5444, -20.0434) (-44.5192, -20.0434) knots 0 0 0 1 1 1
  spline S57 degree 2 poles (-44.489, -21.144) (-44.7855, -21.144) (-45.2378, -21.5209) (-45.4791, -22.4406) (-45.4791, -23.3251) knots 0 0 0 1 2 3 3 3
  spline S58 degree 2 poles (-45.4791, -23.3251) (-45.4791, -24.481) (-44.9313, -25.3655) (-44.489, -25.3655) knots 0 0 0 1 2 2 2
  spline S59 degree 2 poles (-44.489, -25.3655) (-44.0669, -25.3655) (-43.8206, -24.9484) knots 0 0 0 1 1 1
  spline S60 degree 2 poles (-43.8206, -24.9484) (-43.5191, -24.4408) (-43.5191, -23.2548) knots 0 0 0 1 1 1
  spline S61 degree 2 poles (-43.5191, -23.2548) (-43.5191, -22.0537) (-44.0618, -21.144) (-44.489, -21.144) knots 0 0 0 1 2 2 2
  line L48 (-39.6645, -20.0434) -> (-38.6795, -20.5359)
  line L49 (-38.6795, -20.5359) -> (-39.7399, -22.6115)
  spline S62 degree 2 poles (-39.7399, -22.6115) (-38.9659, -22.6115) (-37.8804, -23.7221) (-37.8804, -24.5413) knots 0 0 0 1 2 2 2
  spline S63 degree 2 poles (-37.8804, -24.5413) (-37.8804, -25.3353) (-38.9961, -26.441) (-39.7801, -26.441) knots 0 0 0 1 2 2 2
  spline S64 degree 2 poles (-39.7801, -26.441) (-40.6093, -26.441) (-41.7049, -25.2951) (-41.7049, -24.5564) knots 0 0 0 1 2 2 2
  spline S65 degree 2 poles (-41.7049, -24.5564) (-41.7049, -24.2749) (-41.534, -23.7071) (-41.2274, -23.114) knots 0 0 0 1 2 2 2
  line L50 (-41.2274, -23.114) -> (-39.6645, -20.0434)
  spline S66 degree 2 poles (-39.8052, -23.7121) (-40.1319, -23.7121) (-40.5691, -24.1795) (-40.5691, -24.5262) knots 0 0 0 1 2 2 2
  spline S67 degree 2 poles (-40.5691, -24.5262) (-40.5691, -24.878) (-40.1118, -25.3554) (-39.8052, -25.3554) knots 0 0 0 1 2 2 2
  spline S68 degree 2 poles (-39.8052, -25.3554) (-39.4785, -25.3554) (-39.0162, -24.8881) (-39.0162, -24.5262) knots 0 0 0 1 2 2 2
  spline S69 degree 2 poles (-39.0162, -24.5262) (-39.0162, -24.1795) (-39.4685, -23.7121) (-39.8052, -23.7121) knots 0 0 0 1 2 2 2
  line L51 (-34.5485, -20.0434) -> (-33.3976, -20.0434)
  line L52 (-33.3976, -20.0434) -> (-33.3976, -23.9634)
  line L53 (-33.3976, -23.9634) -> (-32.8549, -23.9634)
  line L54 (-32.8549, -23.9634) -> (-32.8549, -25.0388)
  line L55 (-32.8549, -25.0388) -> (-33.3976, -25.0388)
  line L56 (-33.3976, -25.0388) -> (-33.3976, -26.2902)
  line L57 (-33.3976, -26.2902) -> (-34.5334, -26.2902)
  line L58 (-34.5334, -26.2902) -> (-34.5334, -25.0388)
  line L59 (-34.5334, -25.0388) -> (-37.1919, -25.0388)
  line L60 (-37.1919, -25.0388) -> (-37.1919, -23.9634)
  line L61 (-37.1919, -23.9634) -> (-34.5485, -20.0434)
  line L62 (-34.5334, -23.9634) -> (-34.5334, -21.923)
  line L63 (-34.5334, -21.923) -> (-35.9255, -23.9634)
  line L64 (-35.9255, -23.9634) -> (-34.5334, -23.9634)
  line L65 (-31.1964, -20.1942) -> (-28.3419, -20.1942)
  line L66 (-28.3419, -20.1942) -> (-28.3419, -21.2697)
  line L67 (-28.3419, -21.2697) -> (-30.332, -21.2697)
  line L68 (-30.332, -21.2697) -> (-30.5783, -22.3753)
  spline S70 degree 2 poles (-30.5783, -22.3753) (-30.4727, -22.3451) (-30.2767, -22.315) (-30.1863, -22.315) knots 0 0 0 1 2 2 2
  spline S71 degree 2 poles (-30.1863, -22.315) (-29.3571, -22.315) (-28.2565, -23.4457) (-28.2565, -24.3302) knots 0 0 0 1 2 2 2
  spline S72 degree 2 poles (-28.2565, -24.3302) (-28.2565, -25.2198) (-29.4727, -26.441) (-30.3421, -26.441) knots 0 0 0 1 2 2 2
  spline S73 degree 2 poles (-30.3421, -26.441) (-31.121, -26.441) (-32.2367, -25.5565) (-32.4126, -24.7876) knots 0 0 0 1 2 2 2
  line L69 (-32.4126, -24.7876) -> (-31.1964, -24.7876)
  spline S74 degree 2 poles (-31.1964, -24.7876) (-31.0557, -25.074) (-30.5934, -25.3655) (-30.3169, -25.3655) knots 0 0 0 1 2 2 2
  spline S75 degree 2 poles (-30.3169, -25.3655) (-29.93, -25.3655) (-29.3922, -24.8127) (-29.3922, -24.3755) knots 0 0 0 1 2 2 2
  spline S76 degree 2 poles (-29.3922, -24.3755) (-29.3922, -23.9533) (-29.8948, -23.4106) (-30.2516, -23.4106) knots 0 0 0 1 2 2 2
  spline S77 degree 2 poles (-30.2516, -23.4106) (-30.4426, -23.4106) (-30.8095, -23.6015) (-30.9853, -23.7925) knots 0 0 0 1 2 2 2
  line L70 (-30.9853, -23.7925) -> (-31.9352, -23.5814)
  line L71 (-31.9352, -23.5814) -> (-31.1964, -20.1942)
  spline S78 degree 2 poles (-25.5025, -20.0434) (-24.8341, -20.0434) (-23.8692, -20.6968) (-23.3415, -22.0436) (-23.3415, -23.2447) knots 0 0 0 1 2 3 3 3
  spline S79 degree 2 poles (-23.3415, -23.2447) (-23.3415, -24.4559) (-23.8742, -25.8077) (-24.7788, -26.441) (-25.4673, -26.441) knots 0 0 0 1 2 3 3 3
  spline S80 degree 2 poles (-25.4673, -26.441) (-26.1558, -26.441) (-27.0905, -25.8027) (-27.6232, -24.5011) (-27.6232, -23.3) knots 0 0 0 1 2 3 3 3
  spline S81 degree 2 poles (-27.6232, -23.3) (-27.6232, -21.6265) (-27.1056, -20.8726) knots 0 0 0 1 1 1
  spline S82 degree 2 poles (-27.1056, -20.8726) (-26.5277, -20.0434) (-25.5025, -20.0434) knots 0 0 0 1 1 1
  spline S83 degree 2 poles (-25.4723, -21.144) (-25.7688, -21.144) (-26.2211, -21.5209) (-26.4623, -22.4406) (-26.4623, -23.3251) knots 0 0 0 1 2 3 3 3
  spline S84 degree 2 poles (-26.4623, -23.3251) (-26.4623, -24.481) (-25.9146, -25.3655) (-25.4723, -25.3655) knots 0 0 0 1 2 2 2
  spline S85 degree 2 poles (-25.4723, -25.3655) (-25.0502, -25.3655) (-24.8039, -24.9484) knots 0 0 0 1 1 1
  spline S86 degree 2 poles (-24.8039, -24.9484) (-24.5024, -24.4408) (-24.5024, -23.2548) knots 0 0 0 1 1 1
  spline S87 degree 2 poles (-24.5024, -23.2548) (-24.5024, -22.0537) (-25.0451, -21.144) (-25.4723, -21.144) knots 0 0 0 1 2 2 2
  spline S88 degree 2 poles (-20.7483, -20.0434) (-20.0799, -20.0434) (-19.115, -20.6968) (-18.5873, -22.0436) (-18.5873, -23.2447) knots 0 0 0 1 2 3 3 3
  spline S89 degree 2 poles (-18.5873, -23.2447) (-18.5873, -24.4559) (-19.12, -25.8077) (-20.0246, -26.441) (-20.7131, -26.441) knots 0 0 0 1 2 3 3 3
  spline S90 degree 2 poles (-20.7131, -26.441) (-21.4016, -26.441) (-22.3364, -25.8027) (-22.8691, -24.5011) (-22.8691, -23.3) knots 0 0 0 1 2 3 3 3
  spline S91 degree 2 poles (-22.8691, -23.3) (-22.8691, -21.6265) (-22.3514, -20.8726) knots 0 0 0 1 1 1
  spline S92 degree 2 poles (-22.3514, -20.8726) (-21.7735, -20.0434) (-20.7483, -20.0434) knots 0 0 0 1 1 1
  spline S93 degree 2 poles (-20.7181, -21.144) (-21.0146, -21.144) (-21.4669, -21.5209) (-21.7082, -22.4406) (-21.7082, -23.3251) knots 0 0 0 1 2 3 3 3
  spline S94 degree 2 poles (-21.7082, -23.3251) (-21.7082, -24.481) (-21.1604, -25.3655) (-20.7181, -25.3655) knots 0 0 0 1 2 2 2
  spline S95 degree 2 poles (-20.7181, -25.3655) (-20.296, -25.3655) (-20.0497, -24.9484) knots 0 0 0 1 1 1
  spline S96 degree 2 poles (-20.0497, -24.9484) (-19.7482, -24.4408) (-19.7482, -23.2548) knots 0 0 0 1 1 1
  spline S97 degree 2 poles (-19.7482, -23.2548) (-19.7482, -22.0537) (-20.291, -21.144) (-20.7181, -21.144) knots 0 0 0 1 2 2 2
  line L72 (-16.954, -20.1942) -> (-15.2202, -20.1942)
  line L73 (-15.2202, -20.1942) -> (-15.2202, -26.2902)
  line L74 (-15.2202, -26.2902) -> (-16.371, -26.2902)
  line L75 (-16.371, -26.2902) -> (-16.371, -21.2847)
  line L76 (-16.371, -21.2847) -> (-17.6274, -21.2847)
  line L77 (-17.6274, -21.2847) -> (-16.954, -20.1942)
  point P0 (0, 0)
  point P1 (33.375, 39.75)
  point P2 (33.375, 37.9215)
  point P3 (-33.375, -39.75)
  point P4 (-33.375, -37.9215)
  dimension "d0" = 79.5
  dimension "d27" = 0
  dimension "d28" = 0
  constraints: 4 midpoint, 4 other
  measures "d27" horizontal distance of point (33.375, 39.75) point (33.375, 37.921)
  measures "d28" horizontal distance of point (-33.375, -39.75) point (-33.375, -37.921)
sketch "Sketch8" plane through (0, 0, 0) normal (-1, 0, 0) x (0, 0, 1)
  line L0 (15.0259, -8.5629) -> (51.7241, -8.5629) construction
  line L1 (51.7241, -8.5629) -> (51.7241, -38.6205) construction
  line L2 (51.7241, -38.6205) -> (15.0259, -38.6205) construction
  line L3 (15.0259, -38.6205) -> (15.0259, -8.5629) construction
  line L4 (63.5, -39.75) -> (3.25, -39.75) projected
  line L5 (16.2303, -16.873) -> (15.1146, -16.873)
  spline S0 degree 2 poles (15.1146, -16.873) (15.2001, -16.1996) (15.5971, -15.7875) knots 0 0 0 1 1 1
  spline S1 degree 2 poles (15.5971, -15.7875) (16.1549, -15.2145) (16.9942, -15.2145) knots 0 0 0 1 1 1
  spline S2 degree 2 poles (16.9942, -15.2145) (17.743, -15.2145) (18.7582, -16.1694) (18.7582, -16.8227) knots 0 0 0 1 2 2 2
  spline S3 degree 2 poles (18.7582, -16.8227) (18.7582, -17.2298) (18.3159, -17.8982) (17.8938, -18.1042) knots 0 0 0 1 2 2 2
  spline S4 degree 2 poles (17.8938, -18.1042) (18.4466, -18.2701) (19.0748, -19.0943) (19.0748, -19.6521) knots 0 0 0 1 2 2 2
  spline S5 degree 2 poles (19.0748, -19.6521) (19.0748, -20.4713) (17.8636, -21.6121) (16.9289, -21.6121) knots 0 0 0 1 2 2 2
  spline S6 degree 2 poles (16.9289, -21.6121) (16.0393, -21.6121) (14.9237, -20.5366) (14.8684, -19.6119) knots 0 0 0 1 2 2 2
  line L6 (14.8684, -19.6119) -> (16.0142, -19.6119)
  spline S7 degree 2 poles (16.0142, -19.6119) (16.0896, -20.0843) (16.5972, -20.5467) (16.9892, -20.5467) knots 0 0 0 1 2 2 2
  spline S8 degree 2 poles (16.9892, -20.5467) (17.3962, -20.5467) (17.929, -20.024) (17.929, -19.6471) knots 0 0 0 1 2 2 2
  spline S9 degree 2 poles (17.929, -19.6471) (17.929, -19.235) (17.2053, -18.6671) (16.5268, -18.657) knots 0 0 0 1 2 2 2
  line L7 (16.5268, -18.657) -> (16.5268, -17.662)
  spline S10 degree 2 poles (16.5268, -17.662) (16.949, -17.6268) (17.356, -17.4358) (17.5872, -17.0941) (17.5872, -16.9031) knots 0 0 0 1 2 3 3 3
  spline S11 degree 2 poles (17.5872, -16.9031) (17.5872, -16.6569) (17.2405, -16.3302) (16.959, -16.3302) knots 0 0 0 1 2 2 2
  spline S12 degree 2 poles (16.959, -16.3302) (16.7077, -16.3302) (16.3057, -16.6317) (16.2303, -16.873) knots 0 0 0 1 2 2 2
  spline S13 degree 2 poles (21.7283, -15.2145) (22.3967, -15.2145) (23.3616, -15.8679) (23.8893, -17.2147) (23.8893, -18.4158) knots 0 0 0 1 2 3 3 3
  spline S14 degree 2 poles (23.8893, -18.4158) (23.8893, -19.627) (23.3566, -20.9789) (22.452, -21.6121) (21.7635, -21.6121) knots 0 0 0 1 2 3 3 3
  spline S15 degree 2 poles (21.7635, -21.6121) (21.075, -21.6121) (20.1402, -20.9738) (19.6075, -19.6722) (19.6075, -18.4711) knots 0 0 0 1 2 3 3 3
  spline S16 degree 2 poles (19.6075, -18.4711) (19.6075, -16.7976) (20.1251, -16.0438) knots 0 0 0 1 1 1
  spline S17 degree 2 poles (20.1251, -16.0438) (20.7031, -15.2145) (21.7283, -15.2145) knots 0 0 0 1 1 1
  spline S18 degree 2 poles (21.7584, -16.3151) (21.4619, -16.3151) (21.0096, -16.6921) (20.7684, -17.6117) (20.7684, -18.4962) knots 0 0 0 1 2 3 3 3
  spline S19 degree 2 poles (20.7684, -18.4962) (20.7684, -19.6521) (21.3162, -20.5366) (21.7584, -20.5366) knots 0 0 0 1 2 2 2
  spline S20 degree 2 poles (21.7584, -20.5366) (22.1806, -20.5366) (22.4268, -20.1195) knots 0 0 0 1 1 1
  spline S21 degree 2 poles (22.4268, -20.1195) (22.7284, -19.6119) (22.7284, -18.4259) knots 0 0 0 1 1 1
  spline S22 degree 2 poles (22.7284, -18.4259) (22.7284, -17.2248) (22.1856, -16.3151) (21.7584, -16.3151) knots 0 0 0 1 2 2 2
  line L8 (24.8341, -15.2899) -> (25.9648, -15.2899)
  line L9 (25.9648, -15.2899) -> (25.9648, -16.9534)
  line L10 (25.9648, -16.9534) -> (26.6382, -16.9534)
  line L11 (26.6382, -16.9534) -> (26.6382, -17.9283)
  line L12 (26.6382, -17.9283) -> (25.9648, -17.9283)
  line L13 (25.9648, -17.9283) -> (25.9648, -21.4613)
  line L14 (25.9648, -21.4613) -> (24.8341, -21.4613)
  line L15 (24.8341, -21.4613) -> (24.8341, -17.9283)
  line L16 (24.8341, -17.9283) -> (24.2561, -17.9283)
  line L17 (24.2561, -17.9283) -> (24.2561, -16.9534)
  line L18 (24.2561, -16.9534) -> (24.8341, -16.9534)
  line L19 (24.8341, -16.9534) -> (24.8341, -15.2899)
  line L20 (27.2463, -15.2095) -> (28.367, -15.2095)
  line L21 (28.367, -15.2095) -> (28.367, -17.4107)
  spline S23 degree 2 poles (28.367, -17.4107) (28.6987, -17.1243) (29.3721, -16.8378) (29.7139, -16.8378) knots 0 0 0 1 2 2 2
  spline S24 degree 2 poles (29.7139, -16.8378) (30.3873, -16.8378) (30.8497, -17.3001) knots 0 0 0 1 1 1
  spline S25 degree 2 poles (30.8497, -17.3001) (31.2417, -17.7022) (31.2417, -18.4812) knots 0 0 0 1 1 1
  line L22 (31.2417, -18.4812) -> (31.2417, -21.4613)
  line L23 (31.2417, -21.4613) -> (30.126, -21.4613)
  line L24 (30.126, -21.4613) -> (30.126, -19.4863)
  spline S26 degree 2 poles (30.126, -19.4863) (30.126, -18.7023) (29.9752, -18.1444) (29.6134, -17.8731) (29.352, -17.8731) knots 0 0 0 1 2 3 3 3
  spline S27 degree 2 poles (29.352, -17.8731) (29.0053, -17.8731) (28.5128, -18.3304) (28.4173, -18.7224) knots 0 0 0 1 2 2 2
  spline S28 degree 2 poles (28.4173, -18.7224) (28.367, -18.9234) (28.367, -19.6521) knots 0 0 0 1 1 1
  line L25 (28.367, -19.6521) -> (28.367, -21.4613)
  line L26 (28.367, -21.4613) -> (27.2463, -21.4613)
  line L27 (27.2463, -21.4613) -> (27.2463, -15.2095)
  line L28 (38.0362, -16.1945) -> (37.1768, -16.9534)
  spline S29 degree 2 poles (37.1768, -16.9534) (36.7245, -16.3252) (36.2572, -16.3252) knots 0 0 0 1 1 1
  spline S30 degree 2 poles (36.2572, -16.3252) (36.031, -16.3252) (35.7395, -16.5714) (35.7395, -16.7222) knots 0 0 0 1 2 2 2
  spline S31 degree 2 poles (35.7395, -16.7222) (35.7395, -16.878) (35.8451, -17.0137) knots 0 0 0 1 1 1
  spline S32 degree 2 poles (35.8451, -17.0137) (35.9858, -17.1946) (36.6944, -17.7927) knots 0 0 0 1 1 1
  spline S33 degree 2 poles (36.6944, -17.7927) (37.3527, -18.3505) (37.4934, -18.4962) knots 0 0 0 1 1 1
  spline S34 degree 2 poles (37.4934, -18.4962) (37.8452, -18.853) (38.1417, -19.5013) (38.1417, -19.8833) knots 0 0 0 1 2 2 2
  spline S35 degree 2 poles (38.1417, -19.8833) (38.1417, -20.6371) (37.1065, -21.6121) (36.2722, -21.6121) knots 0 0 0 1 2 2 2
  spline S36 degree 2 poles (36.2722, -21.6121) (35.6239, -21.6121) (34.654, -20.9738) (34.3123, -20.2904) knots 0 0 0 1 2 2 2
  line L29 (34.3123, -20.2904) -> (35.2872, -19.7024)
  spline S37 degree 2 poles (35.2872, -19.7024) (35.7244, -20.5115) (36.2974, -20.5115) knots 0 0 0 1 1 1
  spline S38 degree 2 poles (36.2974, -20.5115) (36.5939, -20.5115) (37.0009, -20.1647) (37.0009, -19.9335) knots 0 0 0 1 2 2 2
  spline S39 degree 2 poles (37.0009, -19.9335) (37.0009, -19.7275) (36.6944, -19.3154) (36.1717, -18.8882) knots 0 0 0 1 2 2 2
  spline S40 degree 2 poles (36.1717, -18.8882) (35.1767, -18.0741) (34.5987, -17.1946) (34.5987, -16.7574) knots 0 0 0 1 2 2 2
  spline S41 degree 2 poles (34.5987, -16.7574) (34.5987, -16.1191) (35.5636, -15.2145) (36.2722, -15.2145) knots 0 0 0 1 2 2 2
  spline S42 degree 2 poles (36.2722, -15.2145) (36.7296, -15.2145) (37.5538, -15.6367) (38.0362, -16.1945) knots 0 0 0 1 2 2 2
  line L30 (43.6397, -19.5315) -> (40.0112, -19.5315)
  spline S43 degree 2 poles (40.0112, -19.5315) (40.0917, -20.0139) (40.7751, -20.5818) (41.3028, -20.5818) knots 0 0 0 1 2 2 2
  spline S44 degree 2 poles (41.3028, -20.5818) (41.936, -20.5818) (42.3934, -20.1396) knots 0 0 0 1 1 1
  line L31 (42.3934, -20.1396) -> (43.3432, -20.5869)
  spline S45 degree 2 poles (43.3432, -20.5869) (42.9864, -21.0894) (41.9913, -21.5769) (41.3078, -21.5769) knots 0 0 0 1 2 2 2
  spline S46 degree 2 poles (41.3078, -21.5769) (40.2474, -21.5769) (38.9157, -20.2401) (38.9157, -19.23) knots 0 0 0 1 2 2 2
  spline S47 degree 2 poles (38.9157, -19.23) (38.9157, -18.1997) (40.2474, -16.8378) (41.2475, -16.8378) knots 0 0 0 1 2 2 2
  spline S48 degree 2 poles (41.2475, -16.8378) (42.313, -16.8378) (43.6447, -18.1997) (43.6447, -19.3154) knots 0 0 0 1 2 2 2
  line L32 (43.6447, -19.3154) -> (43.6397, -19.5315)
  spline S49 degree 2 poles (42.5089, -18.642) (42.3984, -18.2651) (41.74, -17.7977) (41.3028, -17.7977) knots 0 0 0 1 2 2 2
  spline S50 degree 2 poles (41.3028, -17.7977) (40.8304, -17.7977) (40.4736, -18.059) knots 0 0 0 1 1 1
  spline S51 degree 2 poles (40.4736, -18.059) (40.2525, -18.2249) (40.0615, -18.642) knots 0 0 0 1 1 1
  line L33 (40.0615, -18.642) -> (42.5089, -18.642)
  line L34 (45.6851, -16.9534) -> (45.6851, -17.4509)
  spline S52 degree 2 poles (45.6851, -17.4509) (45.9917, -17.1444) (46.7053, -16.8378) (47.1073, -16.8378) knots 0 0 0 1 2 2 2
  spline S53 degree 2 poles (47.1073, -16.8378) (47.9918, -16.8378) (49.2231, -18.1696) (49.2231, -19.2149) knots 0 0 0 1 2 2 2
  spline S54 degree 2 poles (49.2231, -19.2149) (49.2231, -20.22) (47.9466, -21.5769) (47.0772, -21.5769) knots 0 0 0 1 2 2 2
  spline S55 degree 2 poles (47.0772, -21.5769) (46.6852, -21.5769) (46.0168, -21.3005) (45.6851, -20.9839) knots 0 0 0 1 2 2 2
  line L35 (45.6851, -20.9839) -> (45.6851, -23.1097)
  line L36 (45.6851, -23.1097) -> (44.5594, -23.1097)
  line L37 (44.5594, -23.1097) -> (44.5594, -16.9534)
  line L38 (44.5594, -16.9534) -> (45.6851, -16.9534)
  spline S56 degree 2 poles (46.8711, -17.8831) (46.3384, -17.8831) (45.6348, -18.6118) (45.6348, -19.1998) knots 0 0 0 1 2 2 2
  spline S57 degree 2 poles (45.6348, -19.1998) (45.6348, -19.7978) (46.3384, -20.5416) (46.8711, -20.5416) knots 0 0 0 1 2 2 2
  spline S58 degree 2 poles (46.8711, -20.5416) (47.3888, -20.5416) (48.0974, -19.7878) (48.0974, -19.2048) knots 0 0 0 1 2 2 2
  spline S59 degree 2 poles (48.0974, -19.2048) (48.0974, -18.6219) (47.4038, -17.8831) (46.8711, -17.8831) knots 0 0 0 1 2 2 2
  line L39 (50.2986, -15.2899) -> (51.4293, -15.2899)
  line L40 (51.4293, -15.2899) -> (51.4293, -16.9534)
  line L41 (51.4293, -16.9534) -> (52.1027, -16.9534)
  line L42 (52.1027, -16.9534) -> (52.1027, -17.9283)
  line L43 (52.1027, -17.9283) -> (51.4293, -17.9283)
  line L44 (51.4293, -17.9283) -> (51.4293, -21.4613)
  line L45 (51.4293, -21.4613) -> (50.2986, -21.4613)
  line L46 (50.2986, -21.4613) -> (50.2986, -17.9283)
  line L47 (50.2986, -17.9283) -> (49.7206, -17.9283)
  line L48 (49.7206, -17.9283) -> (49.7206, -16.9534)
  line L49 (49.7206, -16.9534) -> (50.2986, -16.9534)
  line L50 (50.2986, -16.9534) -> (50.2986, -15.2899)
  line L51 (25.3442, -27.6921) -> (24.2134, -27.6921)
  spline S60 degree 2 poles (24.2134, -27.6921) (24.2586, -26.7071) (25.4095, -25.5764) (26.3091, -25.5764) knots 0 0 0 1 2 2 2
  spline S61 degree 2 poles (26.3091, -25.5764) (26.8619, -25.5764) (27.7162, -26.0437) (28.2238, -26.9282) (28.2238, -27.3805) knots 0 0 0 1 2 3 3 3
  spline S62 degree 2 poles (28.2238, -27.3805) (28.2238, -27.9233) (27.6057, -29.1747) (26.7815, -30.029) knots 0 0 0 1 2 2 2
  line L52 (26.7815, -30.029) -> (26.098, -30.7477)
  line L53 (26.098, -30.7477) -> (28.2741, -30.7477)
  line L54 (28.2741, -30.7477) -> (28.2741, -31.8231)
  line L55 (28.2741, -31.8231) -> (24.0476, -31.8231)
  line L56 (24.0476, -31.8231) -> (24.0476, -31.2703)
  line L57 (24.0476, -31.2703) -> (25.9372, -29.3455)
  spline S63 degree 2 poles (25.9372, -29.3455) (26.6207, -28.652) (27.073, -27.8127) (27.073, -27.476) knots 0 0 0 1 2 2 2
  spline S64 degree 2 poles (27.073, -27.476) (27.073, -27.1192) (26.6056, -26.6619) (26.2337, -26.6619) knots 0 0 0 1 2 2 2
  spline S65 degree 2 poles (26.2337, -26.6619) (25.8618, -26.6619) (25.3592, -27.2147) (25.3442, -27.6921) knots 0 0 0 1 2 2 2
  spline S66 degree 2 poles (30.9778, -25.5764) (31.6462, -25.5764) (32.6111, -26.2297) (33.1388, -27.5765) (33.1388, -28.7776) knots 0 0 0 1 2 3 3 3
  spline S67 degree 2 poles (33.1388, -28.7776) (33.1388, -29.9888) (32.6061, -31.3407) (31.7015, -31.9739) (31.013, -31.9739) knots 0 0 0 1 2 3 3 3
  spline S68 degree 2 poles (31.013, -31.9739) (30.3245, -31.9739) (29.3897, -31.3356) (28.857, -30.034) (28.857, -28.8329) knots 0 0 0 1 2 3 3 3
  spline S69 degree 2 poles (28.857, -28.8329) (28.857, -27.1594) (29.3747, -26.4056) knots 0 0 0 1 1 1
  spline S70 degree 2 poles (29.3747, -26.4056) (29.9526, -25.5764) (30.9778, -25.5764) knots 0 0 0 1 1 1
  spline S71 degree 2 poles (31.008, -26.677) (30.7115, -26.677) (30.2592, -27.0539) (30.0179, -27.9735) (30.0179, -28.858) knots 0 0 0 1 2 3 3 3
  spline S72 degree 2 poles (30.0179, -28.858) (30.0179, -30.0139) (30.5657, -30.8984) (31.008, -30.8984) knots 0 0 0 1 2 2 2
  spline S73 degree 2 poles (31.008, -30.8984) (31.4301, -30.8984) (31.6764, -30.4813) knots 0 0 0 1 1 1
  spline S74 degree 2 poles (31.6764, -30.4813) (31.9779, -29.9737) (31.9779, -28.7877) knots 0 0 0 1 1 1
  spline S75 degree 2 poles (31.9779, -28.7877) (31.9779, -27.5866) (31.4351, -26.677) (31.008, -26.677) knots 0 0 0 1 2 2 2
  line L58 (34.8525, -27.6921) -> (33.7218, -27.6921)
  spline S76 degree 2 poles (33.7218, -27.6921) (33.767, -26.7071) (34.9178, -25.5764) (35.8174, -25.5764) knots 0 0 0 1 2 2 2
  spline S77 degree 2 poles (35.8174, -25.5764) (36.3702, -25.5764) (37.2246, -26.0437) (37.7322, -26.9282) (37.7322, -27.3805) knots 0 0 0 1 2 3 3 3
  spline S78 degree 2 poles (37.7322, -27.3805) (37.7322, -27.9233) (37.114, -29.1747) (36.2898, -30.029) knots 0 0 0 1 2 2 2
  line L59 (36.2898, -30.029) -> (35.6063, -30.7477)
  line L60 (35.6063, -30.7477) -> (37.7824, -30.7477)
  line L61 (37.7824, -30.7477) -> (37.7824, -31.8231)
  line L62 (37.7824, -31.8231) -> (33.5559, -31.8231)
  line L63 (33.5559, -31.8231) -> (33.5559, -31.2703)
  line L64 (33.5559, -31.2703) -> (35.4455, -29.3455)
  spline S79 degree 2 poles (35.4455, -29.3455) (36.129, -28.652) (36.5813, -27.8127) (36.5813, -27.476) knots 0 0 0 1 2 2 2
  spline S80 degree 2 poles (36.5813, -27.476) (36.5813, -27.1192) (36.1139, -26.6619) (35.742, -26.6619) knots 0 0 0 1 2 2 2
  spline S81 degree 2 poles (35.742, -26.6619) (35.3701, -26.6619) (34.8676, -27.2147) (34.8525, -27.6921) knots 0 0 0 1 2 2 2
  line L65 (39.5464, -25.7271) -> (42.4009, -25.7271)
  line L66 (42.4009, -25.7271) -> (42.4009, -26.8026)
  line L67 (42.4009, -26.8026) -> (40.4108, -26.8026)
  line L68 (40.4108, -26.8026) -> (40.1645, -27.9082)
  spline S82 degree 2 poles (40.1645, -27.9082) (40.2701, -27.8781) (40.4661, -27.8479) (40.5565, -27.8479) knots 0 0 0 1 2 2 2
  spline S83 degree 2 poles (40.5565, -27.8479) (41.3857, -27.8479) (42.4863, -28.9787) (42.4863, -29.8632) knots 0 0 0 1 2 2 2
  spline S84 degree 2 poles (42.4863, -29.8632) (42.4863, -30.7527) (41.2701, -31.9739) (40.4007, -31.9739) knots 0 0 0 1 2 2 2
  spline S85 degree 2 poles (40.4007, -31.9739) (39.6218, -31.9739) (38.5061, -31.0894) (38.3302, -30.3205) knots 0 0 0 1 2 2 2
  line L69 (38.3302, -30.3205) -> (39.5464, -30.3205)
  spline S86 degree 2 poles (39.5464, -30.3205) (39.6871, -30.6069) (40.1495, -30.8984) (40.4259, -30.8984) knots 0 0 0 1 2 2 2
  spline S87 degree 2 poles (40.4259, -30.8984) (40.8128, -30.8984) (41.3506, -30.3456) (41.3506, -29.9084) knots 0 0 0 1 2 2 2
  spline S88 degree 2 poles (41.3506, -29.9084) (41.3506, -29.4862) (40.848, -28.9435) (40.4912, -28.9435) knots 0 0 0 1 2 2 2
  spline S89 degree 2 poles (40.4912, -28.9435) (40.3002, -28.9435) (39.9334, -29.1344) (39.7575, -29.3254) knots 0 0 0 1 2 2 2
  line L70 (39.7575, -29.3254) -> (38.8076, -29.1143)
  line L71 (38.8076, -29.1143) -> (39.5464, -25.7271)
  point P0 (0, 0)
  point P1 (33.375, -39.75)
  point P2 (33.375, -38.6205)
  dimension "d0" = 79.5
  dimension "d29" = 0
  constraints: 2 midpoint, 2 other
  measures "d29" horizontal distance of point (33.375, -39.75) point (33.375, -38.62)
emboss "Emboss1" sketch "Sketch6" operation cut depth 1.5 direction (1, 0, 0)
emboss "Emboss2" sketch "Sketch7" operation cut depth 1.5 direction (1, 0, 0)
emboss "Emboss3" sketch "Sketch8" operation cut depth 1.5 direction (1, 0, 0)
fillet "Fillet1" radius 1 16 edges at (88, 0, 63.5) (0, 0, 63.5) (88, 0, -63.5) (0, 0, -63.5) (44, 39.75, -63.5) (88, 39.75, -33.375) (88, 39.75, 33.375) (44, 39.75, 63.5) (0, 39.75, 33.375) (0, 39.75, -33.375) (0, -39.75, -33.375) (0, -39.75, 33.375) (44, -39.75, 63.5) (88, -39.75, 33.375) (88, -39.75, -33.375) (44, -39.75, -63.5)
body "Solid1"
